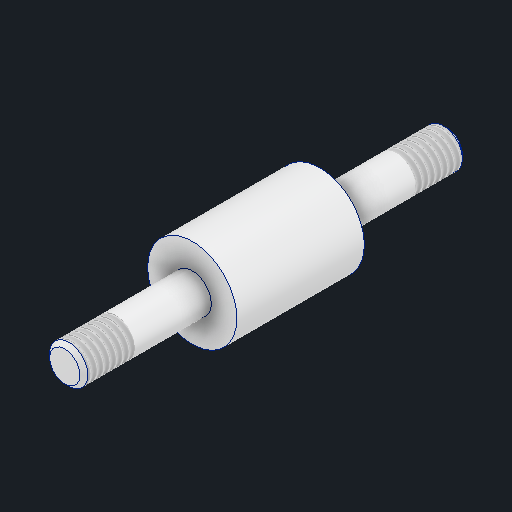
# Autodesk Inventor part: Clavija
Saved by Autodesk Inventor 2025.3 (Build 293356030, 356C)
## iProperties
Created: 2024-11-17
Part Number: Clavija
Material: Aluminio 6061
Document SubType Name: Modeling
Designer: Usuario
Density: 2.7 g/cm^3
Appearance: Aluminio - Plano
Mass: 1.41855 g
Surface Area: 4.81744 cm^2
Volume: 0.525391 cm^3
Author: Usuario
Autodesk Inventor part; units mm, degrees
ref_plane "YZ Plane" through (0, 0, 0) normal (1, 0, 0) x (0, 1, 0)
ref_plane "XZ Plane" through (0, 0, 0) normal (0, 1, 0) x (-1, 0, 0)
ref_plane "XY Plane" through (0, 0, 0) normal (0, 0, 1) x (1, 0, 0)
sketch "Boceto1" plane through (0, 0, 0) normal (0, 1, 0) x (-1, 0, 0)
  line L0 (0, 15) -> (1.5, 15)
  line L1 (1.5, 15) -> (1.5, 5)
  line L2 (1.5, 5) -> (3.5, 5)
  line L3 (3.5, 5) -> (3.5, -5)
  line L4 (3.5, -5) -> (1.5, -5)
  line L5 (1.5, -5) -> (1.5, -15)
  line L6 (1.5, -15) -> (0, -15)
  line L7 (0, -15) -> (0, 15)
  point P0 (0, 0)
  point P1 (0, 0)
  dimension "d0" = 7
  dimension "d1" = 3
  dimension "Dedos" = 10
  dimension "d3" = 30
  constraints: 16 end point, 6 perpendicular, 2 point on line, 1 coincident, 1 collinear, 1 horizontal, 1 midpoint, 1 vertical alignment
  measures "d0" diameter of L3 L7
  measures "d1" diameter of L1 L7
  measures "Dedos" distance of L2.end L3.end
  measures "d3" distance between parallel lines of L6 L0
revolve "Revolución1" add sketch "Boceto1" angle 360 about axis through (0, 0, -15) along (0, 0, 1)
thread "Rosca2" size "M3x0.5" class "6g" standard "ANSI Metric M Profile" length 4
thread "Rosca3" size "M3x0.5" class "6g" standard "ANSI Metric M Profile" length 4 offset 6
chamfer "Chaflán1" distance 0.3067 angle 45 2 edges at (1.5, 0, 15) (1.5, 0, -15)
